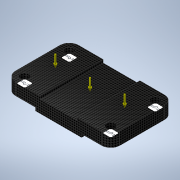
# Autodesk Inventor part: topPlate
Saved by Autodesk Inventor 2020 (Build 240168000, 168)
## iProperties
Created: 2021-06-13
Part Number: topPlate
Material: Iron, Malleable
Document SubType Name: Modeling
Designer: joelm
Density: 7.15 g/cm^3
Appearance: Skid Plate
Mass: 1246.3 g
Surface Area: 315.626 cm^2
Volume: 174.308 cm^3
Author: joelm
Autodesk Inventor part; units mm, degrees
ref_plane "YZ Plane" through (0, 0, 0) normal (1, 0, 0) x (0, 1, 0)
ref_plane "XZ Plane" through (0, 0, 0) normal (0, 1, 0) x (-1, 0, 0)
ref_plane "XY Plane" through (0, 0, 0) normal (0, 0, 1) x (1, 0, 0)
sketch "Sketch1" plane through (0, 0, 0) normal (0, 0, 1) x (1, 0, 0)
  line L0 (0, 0) -> (30, 0)
  line L1 (30, 0) -> (30, 4)
  line L2 (30, 4) -> (68, 4)
  line L3 (68, 4) -> (68, 20)
  line L4 (68, 20) -> (24, 20)
  line L5 (24, 20) -> (24, 16)
  line L6 (24, 16) -> (0, 16)
  line L7 (0, 16) -> (0, 0)
  dimension "d0" = 30
  dimension "d1" = 4
  dimension "d2" = 38
  dimension "d3" = 16
  dimension "d4" = 44
  dimension "d5" = 4
  constraints: 16 end point, 6 perpendicular, 1 horizontal, 1 vertical
  measures "d0" distance of L0.start L0.end
  measures "d1" distance of L0.end L1.end
  measures "d2" distance of L1.end L2.end
  measures "d3" distance of L2.end L3.end
  measures "d4" distance of L3.end L4.end
  measures "d5" distance of L4.end L5.end
extrude "Extrusion1" add sketch "Sketch1" against normal blind 82
sketch "Sketch2" plane through (24, 20, 0) normal (0, 1, 0) x (1, 0, 0)
  circle A0 centre (32, 12) radius 5.5
  circle A1 centre (32, 70) radius 5.5
  line L0 (44, 0) -> (44, 82) projected
  line L1 (44, 0) -> (0, 0) projected
  line L2 (0, 82) -> (44, 82) projected
  point P0 (-24, 0)
  dimension "d8" = 11
  dimension "d9" = 11
  dimension "d10" = 12
  dimension "d11" = 12
  dimension "d12" = 12
  dimension "d13" = 12
  constraints: 2 centre point
  measures "d8" diameter of A0
  measures "d9" diameter of A1
  measures "d10" distance from line of L0 A0.centre
  measures "d11" distance from line of L1 A0.centre
  measures "d12" distance from line of L2 A1.centre
  measures "d13" distance from line of L0 A1.centre
extrude "Extrusion2" cut sketch "Sketch2" against normal blind 82 contours A0
extrude "Extrusion3" cut sketch "Sketch2" against normal blind 82 contours A1
fillet "Fillet1" radius 12 1 edges at (68, 12, 0)
fillet "Fillet2" radius 12 1 edges at (68, 12, -82)
mirror "Mirror1" about plane through (0, 0, 0) normal (1, 0, 0) of "Extrusion1", "Fillet1", "Extrusion2", "Extrusion3", "Fillet2"
body "Solid1"
